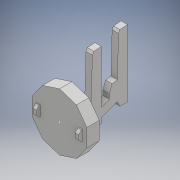
# Autodesk Inventor part: doomba
Saved by Autodesk Inventor 2018 (Build 220112000, 112)
## iProperties
Created: 2020-02-15
Part Number: doomba
Material: Generic
Document SubType Name: Modeling
Designer: TestUser
Density: 1 g/cm^3
Appearance: Default
Author: TestUser
Autodesk Inventor part; units mm, degrees
ref_plane "YZ Plane" through (0, 0, 0) normal (1, 0, 0) x (0, 1, 0)
ref_plane "XZ Plane" through (0, 0, 0) normal (0, 1, 0) x (-1, 0, 0)
ref_plane "XY Plane" through (0, 0, 0) normal (0, 0, 1) x (1, 0, 0)
sketch "Sketch1" plane through (0, 0, 0) normal (0, 1, 0) x (-1, 0, 0)
  line L0 (0, -180) -> (-105.8013, -145.6231)
  line L1 (-105.8013, -145.6231) -> (-171.1902, -55.6231)
  line L2 (-171.1902, -55.6231) -> (-171.1902, 55.6231)
  line L3 (-171.1902, 55.6231) -> (-105.8013, 145.6231)
  line L4 (-105.8013, 145.6231) -> (0, 180)
  line L5 (0, 180) -> (105.8013, 145.6231)
  line L6 (105.8013, 145.6231) -> (171.1902, 55.6231)
  line L7 (171.1902, 55.6231) -> (171.1902, -55.6231)
  line L8 (171.1902, -55.6231) -> (105.8013, -145.6231)
  line L9 (105.8013, -145.6231) -> (0, -180)
  point P0 (0, 0)
  dimension "d12" = 360
  dimension "d13" = 0
  constraints: 20 end point, 21 other
  measures "d12" distance of L0.start L4.end
  measures "d13" horizontal distance of point (0, 0) L4.end
extrude "Extrusion1" add sketch "Sketch1" along normal blind 77.75
sketch "Sketch2" plane through (0, 0, 0) normal (0, -1, 0) x (1, 0, 0)
  line L0 (143.5508, -32.8086) -> (121.9699, -32.8086)
  line L1 (121.9699, -32.8086) -> (121.9699, 32.445)
  line L2 (121.9699, 32.445) -> (143.5508, 32.445)
  line L3 (143.5508, 32.445) -> (143.5508, -32.8086)
  line L4 (0, 0) -> (0, -59.4924)
  constraints: 10 end point, 2 parallel, 1 horizontal, 1 perpendicular, 1 vertical
extrude "Extrusion2" add sketch "Sketch2" along normal blind 36.75
chamfer "Chamfer1" distance 17.75 angle 45 2 edges at (132.7603, -36.75, 32.445) (132.7603, -36.75, -32.8086)
mirror "Mirror1" about plane through (0, 0, 0) normal (1, 0, 0) of "Extrusion2", "Chamfer1"
move faces "Move1" translate (0, 13, 0) faces at (129.1635, -30.8333, 20.6117) (129.1635, -12.6667, 32.445) (121.9699, -12.25, -5.1407) (129.1635, -36.75, 4.7772) (136.3571, -30.8333, -20.9753) (136.3571, -12.6667, -32.8086) (143.5508, -12.25, 4.7772)
move faces "Move2" translate (0, 14, 0) faces at (-143.5508, -12.25, 4.7772) (-129.1635, -30.8333, 20.6117) (-129.1635, -36.75, 4.7772) (-136.3571, -30.8333, -20.9753) (-129.1635, -12.6667, 32.445) (-121.9699, -12.25, -5.1407) (-136.3571, -12.6667, -32.8086)
sketch "Sketch3" plane through (0, 77.75, 0) normal (0, 1, 0) x (1, 0, 0)
  line L0 (9.7495, -156.4565) -> (1.3382, -160.0591)
  line L1 (1.3382, -160.0591) -> (-7.5842, -158.0297)
  line L2 (-7.5842, -158.0297) -> (-13.6097, -151.1434)
  line L3 (-13.6097, -151.1434) -> (-14.4368, -142.0305)
  line L4 (-14.4368, -142.0305) -> (-9.7495, -134.1719)
  line L5 (-9.7495, -134.1719) -> (-1.3382, -130.5692)
  line L6 (-1.3382, -130.5692) -> (7.5842, -132.5987)
  line L7 (7.5842, -132.5987) -> (13.6097, -139.485)
  line L8 (13.6097, -139.485) -> (14.4368, -148.5979)
  line L9 (14.4368, -148.5979) -> (9.7495, -156.4565)
  point P0 (0, 0)
  point P1 (0, -145.3142)
  constraints: 20 end point, 21 other
extrude "Extrusion3" add sketch "Sketch3" along normal blind 10.5
sketch "Sketch6" plane through (0, 0, 0) normal (1, 0, 0) x (0, 1, 0)
  line L0 (77.75, -145.6231) -> (77.75, -55.6231) projected
  line L1 (77.75, -123.89) -> (176.7699, -87.6295)
  line L2 (176.7699, -87.6295) -> (194.9001, -120.1129)
  line L3 (194.9001, -120.1129) -> (241.7366, -120.1129)
  line L4 (241.7366, 299.9045) -> (194.9001, 296.1274)
  line L5 (194.9001, 296.1274) -> (185.835, 279.508)
  line L6 (178.2267, 19.5558) -> (148.7448, 20.4187)
  line L7 (148.7448, 20.4187) -> (132.1997, -21.152)
  line L8 (132.1997, -21.152) -> (131.4487, -46.8134)
  line L9 (177.0352, -21.152) -> (152.4262, -21.152)
  line L10 (152.4262, -21.152) -> (145.5289, -8.7942)
  line L11 (145.5289, -8.7942) -> (152.4262, -4.9445)
  line L12 (152.4262, -4.9445) -> (157.5524, -14.1289)
  line L13 (157.5524, -14.1289) -> (177.2874, -12.5374)
  line L14 (127.26, -48.3473) -> (127.26, -17.7195)
  line L15 (127.26, -17.7195) -> (145.1746, 27.2923)
  line L16 (145.1746, 27.2923) -> (178.5742, 31.4309)
  line L17 (185.835, 279.508) -> (178.5742, 31.4309)
  line L18 (178.2267, 19.5558) -> (177.2874, -12.5374)
  line L19 (177.0352, -21.152) -> (176.7699, -30.2171)
  line L20 (176.7699, -30.2171) -> (131.4487, -46.8134)
  line L21 (127.26, -48.3473) -> (77.75, -66.4776)
  line L22 (241.7366, -87.6295) -> (340.7565, -51.369)
  line L23 (340.7565, -51.369) -> (358.8868, -83.8524)
  line L24 (358.8868, -83.8524) -> (405.7232, -83.8524)
  line L25 (405.7232, -83.8524) -> (405.7232, 336.165)
  line L26 (405.7232, 336.165) -> (358.8868, 332.3878)
  line L27 (358.8868, 332.3878) -> (349.8216, 315.7685)
  line L28 (342.2133, 55.8163) -> (312.7314, 56.6792)
  line L29 (312.7314, 56.6792) -> (296.1863, 15.1085)
  line L30 (296.1863, 15.1085) -> (295.4353, -10.553)
  line L31 (341.0218, 15.1085) -> (316.4128, 15.1085)
  line L32 (316.4128, 15.1085) -> (309.5155, 27.4663)
  line L33 (309.5155, 27.4663) -> (316.4128, 31.316)
  line L34 (316.4128, 31.316) -> (321.539, 22.1316)
  line L35 (321.539, 22.1316) -> (341.274, 23.7231)
  line L36 (291.2466, -12.0868) -> (291.2466, 18.541)
  line L37 (291.2466, 18.541) -> (309.1613, 63.5528)
  line L38 (309.1613, 63.5528) -> (342.5609, 67.6914)
  line L39 (349.8216, 315.7685) -> (342.5609, 67.6914)
  line L40 (342.2133, 55.8163) -> (341.274, 23.7231)
  line L41 (341.0218, 15.1085) -> (340.7565, 6.0434)
  line L42 (340.7565, 6.0434) -> (295.4353, -10.553)
  line L43 (291.2466, -12.0868) -> (241.7366, -30.2171)
  line L44 (241.7366, -120.1129) -> (241.7366, -87.6295)
  line L45 (241.7366, -30.2171) -> (241.7366, 299.9045)
  point P0 (0, 0)
  constraints: 90 end point, 15 perpendicular, 10 parallel, 2 horizontal, 2 point on line, 2 vertical
extrude "Extrusion5" add sketch "Sketch6" along normal blind 20 and the other way blind 20 contours L0 L21 L14 L15 L16 L17 L5 L4 L45 L43 L36 L37 L38 L39 L27 L26 L25 L24 L23 L22 L44 L3 L2 L1 | L40 L35 L34 L33 L32 L31 L41 L42 L30 L29 L28
sketch "Sketch7" plane through (0, 0, 0) normal (0, 0, 1) x (1, 0, 0)
  point P0 (0, 0)
body "Solid1"
